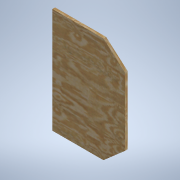
# Autodesk Inventor part: Slope
Saved by Autodesk Inventor 2020 (Build 240168000, 168)
## iProperties
Created: 2020-01-25
Part Number: Slope
Material: Wood (Oak)
Document SubType Name: Modeling
Designer: 1cikaychapman
Density: 0.76 g/cm^3
Appearance: Plywood - Weathered
Author: 1cikaychapman
Autodesk Inventor part; units mm, degrees
ref_plane "YZ Plane" through (0, 0, 0) normal (1, 0, 0) x (0, 1, 0)
ref_plane "XZ Plane" through (0, 0, 0) normal (0, 1, 0) x (-1, 0, 0)
ref_plane "XY Plane" through (0, 0, 0) normal (0, 0, 1) x (1, 0, 0)
sketch "Sketch1" plane through (0, 0, 0) normal (0, 0, 1) x (1, 0, 0)
  line L0 (0, 0) -> (241.3, 0)
  line L1 (0, 497.84) -> (0, 0)
  line L2 (241.3, 0) -> (342.9, 88.9)
  line L3 (342.9, 88.9) -> (342.9, 408.94)
  line L4 (241.3, 497.84) -> (342.9, 408.94)
  line L5 (241.3, 497.84) -> (0, 497.84)
  dimension "d9" = 342.9
  dimension "d10" = 88.9
  dimension "d11" = 88.9
  dimension "d13" = 101.6
  dimension "d14" = 101.6
  constraints: 12 end point, 2 parallel, 1 horizontal, 1 perpendicular
  measures "d9" distance between parallel lines of L3 L1
  measures "d10" vertical distance of L0.end L2.end
  measures "d11" vertical distance of L4.start L3.end
  measures "d13" horizontal distance of L2.end L0.end
  measures "d14" horizontal distance of L3.end L4.start
extrude "Extrusion1" add sketch "Sketch1" along normal blind 12.7
body "Solid1"
